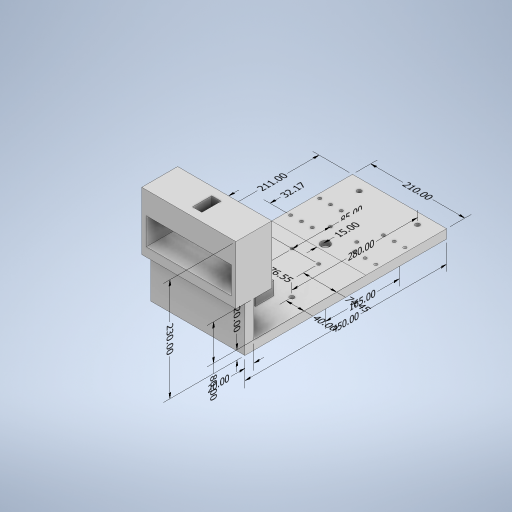
# Autodesk Inventor part: base
Saved by Autodesk Inventor 2023 (Build 270158000, 158)
## iProperties
Created: 2022-07-03
Part Number: base
Material: Genérico
Document SubType Name: Modeling
Designer: inigo
Density: 1 g/cm^3
Appearance: Valor por defecto
Author: inigo
Autodesk Inventor part; units mm, degrees
ref_plane "YZ Plane" through (0, 0, 0) normal (1, 0, 0) x (0, 1, 0)
ref_plane "XZ Plane" through (0, 0, 0) normal (0, 1, 0) x (-1, 0, 0)
ref_plane "XY Plane" through (0, 0, 0) normal (0, 0, 1) x (1, 0, 0)
sketch "Boceto1" plane through (0, 0, 0) normal (1, 0, 0) x (0, 1, 0)
  line L0 (10, 225) -> (-10, 225)
  line L1 (-10, 225) -> (-10, -225)
  line L2 (-10, -225) -> (10, -225)
  line L3 (10, -225) -> (10, 225)
  line L4 (10, 225) -> (-10, -225) construction
  line L5 (-10, 225) -> (10, -225) construction
  point P0 (0, 0)
  dimension "d0" = 20
  dimension "d1" = 450
  constraints: 12 end point, 2 midpoint, 2 parallel, 1 horizontal, 1 perpendicular
  measures "d0" distance of L2.end L1.end
  measures "d1" distance of L1.end L0.end
extrude "Extrusión1" add sketch "Boceto1" along normal blind 210
sketch "Boceto2" plane through (0, 10, 225) normal (0, 1, 0) x (1, 0, 0)
  line L0 (0, 0) -> (0, 450) projected
  line L1 (210, 0) -> (210, 450) projected
  line L2 (0, 0) -> (210, 0)
  line L3 (210, 0) -> (210, 20)
  line L4 (210, 20) -> (0, 20)
  line L5 (0, 20) -> (0, 0)
  point P0 (0, 225)
  dimension "d4" = 20
  constraints: 8 end point, 2 parallel, 1 horizontal, 1 perpendicular, 1 point on line
  measures "d4" distance of L3.end L2.end
extrude "Extrusión2" add sketch "Boceto2" along normal blind 80
sketch "Boceto3" plane through (0, 90, 225) normal (0, 1, 0) x (1, 0, 0)
  line L0 (0, 0) -> (210, 0) projected
  line L1 (0, 0) -> (210, 0)
  line L2 (210, 0) -> (210, -20)
  line L3 (210, -20) -> (0, -20)
  line L4 (0, -20) -> (0, 0)
  line L5 (0, 0) -> (210, 0)
  line L6 (210, 0) -> (210, 60)
  line L7 (210, 60) -> (0, 60)
  line L8 (0, 60) -> (0, 0)
  point P0 (0, 225)
  dimension "d7" = 20
  dimension "d8" = 210
  dimension "d9" = 60
  constraints: 16 end point, 4 parallel, 2 horizontal, 2 perpendicular
  measures "d7" distance of L1.end L2.end
  measures "d8" distance of L7.end L6.end
  measures "d9" distance of L6.end L5.end
extrude "Extrusión3" add sketch "Boceto3" along normal blind 130
sketch "Boceto4" plane through (0, 90, 245) normal (0, 0, 1) x (1, 0, 0)
  line L0 (10, 80) -> (200, 80)
  line L1 (200, 80) -> (200, 20)
  line L2 (200, 20) -> (10, 20)
  line L3 (10, 20) -> (10, 80)
  point P0 (0, -90)
  point P1 (0, 130)
  point P2 (210, 0)
  dimension "d12" = 190
  dimension "d13" = 60
  constraints: 8 end point, 2 parallel, 1 horizontal, 1 perpendicular
  measures "d12" distance of L1.end L2.end
  measures "d13" distance of L0.end L1.end
extrude "Extrusión4" cut sketch "Boceto4" against normal blind 60
sketch "Boceto5" plane through (0, 220, 225) normal (0, 1, 0) x (1, 0, 0)
  line L0 (94.5, -1.5) -> (115.5, -1.5)
  line L1 (115.5, -1.5) -> (115.5, 41.5)
  line L2 (115.5, 41.5) -> (94.5, 41.5)
  line L3 (94.5, 41.5) -> (94.5, -1.5)
  line L4 (94.5, -1.5) -> (115.5, 41.5) construction
  line L5 (115.5, -1.5) -> (94.5, 41.5) construction
  point P0 (0, 225)
  point P1 (105, 20)
  dimension "d18" = 21
  dimension "d19" = 43
  constraints: 12 end point, 2 midpoint, 2 parallel, 1 horizontal, 1 perpendicular
  measures "d18" distance of L2.end L1.end
  measures "d19" distance of L1.end L0.end
extrude "Extrusión5" cut sketch "Boceto5" against normal blind 43
sketch "Boceto6" plane through (0, 10, -225) normal (0, 1, 0) x (1, 0, 0)
  circle A0 centre (40, -305) radius 5
  circle A1 centre (40, -25) radius 5
  circle A2 centre (170, -305) radius 5
  circle A3 centre (170, -25) radius 5
  line L0 (0, -470) -> (210, -470) projected
  line L1 (0, 0) -> (210, 0) projected
  line L2 (0, 0) -> (0, -430) projected
  line L3 (210, 0) -> (210, -430) projected
  point P0 (0, -225)
  dimension "d23" = 10
  dimension "d24" = 10
  dimension "d25" = 10
  dimension "d26" = 10
  dimension "d27" = 165
  dimension "d28" = 25
  dimension "d29" = 25
  dimension "d30" = 165
  dimension "d31" = 40
  dimension "d32" = 40
  dimension "d33" = 40
  dimension "d34" = 40
  constraints: 4 centre point
  measures "d23" diameter of A0
  measures "d24" diameter of A1
  measures "d25" diameter of A2
  measures "d26" diameter of A3
  measures "d27" distance from line of L0 A0.centre
  measures "d28" distance from line of L1 A1.centre
  measures "d29" distance from line of L1 A3.centre
  measures "d30" distance from line of L0 A2.centre
  measures "d31" distance from line of L2 A0.centre
  measures "d32" distance from line of L2 A1.centre
  measures "d33" distance from line of L3 A3.centre
  measures "d34" distance from line of L3 A2.centre
extrude "Extrusión6" cut sketch "Boceto6" against normal blind 43
sketch "Boceto7" plane through (0, 10, -225) normal (0, 1, 0) x (1, 0, 0)
  line L0 (0, 0) -> (210, 0) projected
  line L1 (0, 0) -> (210, 0)
  line L2 (210, 0) -> (105, 0)
  line L3 (210, -390) -> (0, -390) projected
  line L4 (105, -390) -> (105, 0)
  circle A0 centre (40, -305) radius 5 projected
  circle A1 centre (40, -25) radius 5 projected
  line L5 (40, -305) -> (40, -25)
  line L6 (40, -165) -> (169.1036, -165)
  circle A2 centre (104.5518, -165) radius 10
  point P0 (0, -225)
  dimension "d44" = 20
  constraints: 10 end point, 4 midpoint, 2 horizontal, 1 centre point, 1 perpendicular
  measures "d44" diameter of A2
extrude "Extrusión7" cut sketch "Boceto7" against normal blind 10 contours A2 L6 L4 | L4 L6 A2 | L6 A2 L4 | L4 A2 L6
sketch "Boceto8" plane through (0, 10, -225) normal (0, 1, 0) x (1, 0, 0)
  circle A0 centre (104.5518, -165) radius 10 projected
  circle A1 centre (135.5518, -211) radius 3.5
  line L0 (104.5518, -165) -> (126.1125, -165)
  circle A2 centre (135.5518, -126) radius 3.5
  circle A3 centre (76.5518, -126) radius 3.5
  circle A4 centre (76.5518, -211) radius 3.5
  point P0 (0, -225)
  dimension "d51" = 7
  dimension "d52" = 7
  dimension "d54" = 7
  constraints: 4 centre point, 2 end point, 1 horizontal
  measures "d51" diameter of A1
  measures "d52" diameter of A2
  measures "d54" diameter of A4
extrude "Extrusión8" cut sketch "Boceto8" against normal blind 20 contours A1 | A2 | A3 | A4
sketch "Boceto9" plane through (0, 10, -225) normal (0, 1, 0) x (1, 0, 0)
  line L0 (0, -430) -> (210, -430) projected
  line L1 (0, -430) -> (210, -430)
  circle A0 centre (93.5, -410) radius 3
  line L2 (210, -430) -> (0, -430)
  circle A1 centre (116.5, -410) radius 3
  circle A2 centre (93.5, -380) radius 3
  circle A3 centre (116.5, -380) radius 3
  point P0 (0, -225)
  dimension "d59" = 20
  dimension "d64" = 20
  dimension "d65" = 30
  dimension "d66" = 30
  constraints: 4 centre point, 4 end point, 1 collinear
  measures "d59" distance from line of L0 A0.centre
  measures "d64" distance from line of A1.centre L0
  measures "d65" distance between centres of A3 A1
  measures "d66" distance of A2.centre A0.centre
extrude "Extrusión9" cut sketch "Boceto9" against normal blind 20
sketch "Boceto10" plane through (0, 10, -225) normal (0, 1, 0) x (1, 0, 0)
  line L0 (0, -430) -> (210, -430) projected
  line L1 (68, -358.4637) -> (142, -358.4637)
  line L2 (142, -358.4637) -> (68, -358.4637)
  line L3 (68, -358.4637) -> (68, -327.4637)
  line L4 (68, -327.4637) -> (142, -327.4637)
  line L5 (142, -327.4637) -> (142, -358.4637)
  line L6 (68, -358.4637) -> (142, -327.4637)
  line L7 (68, -327.4637) -> (142, -358.4637)
  line L8 (63, -363.4637) -> (147, -363.4637)
  line L9 (147, -363.4637) -> (147, -322.4637)
  line L10 (147, -322.4637) -> (63, -322.4637)
  line L11 (63, -322.4637) -> (63, -363.4637)
  line L12 (63, -363.4637) -> (147, -322.4637) construction
  line L13 (147, -363.4637) -> (63, -322.4637) construction
  point P0 (0, -225)
  point P1 (105, -342.9637)
  dimension "d68" = 74
  dimension "d69" = 31
  dimension "d70" = 84
  dimension "d71" = 41
  constraints: 26 end point, 4 parallel, 3 midpoint, 2 horizontal, 2 perpendicular
  measures "d68" distance of L1.start L1.end
  measures "d69" distance of L2.end L3.end
  measures "d70" distance of L10.end L9.end
  measures "d71" distance of L9.end L8.end
extrude "Extrusión10" cut sketch "Boceto10" against normal blind 10 contours L6 L7 L1 | L3 L7 L6 | L7 L6 L5 | L4 L6 L7
sketch "Boceto11" plane through (0, 10, -225) normal (0, 1, 0) x (1, 0, 0)
  line L0 (142, -358.4637) -> (68, -358.4637) projected
  line L1 (68, -358.4637) -> (142, -327.4637)
  line L2 (68, -327.4637) -> (142, -327.4637) projected
  line L3 (142, -327.4637) -> (68, -327.4637)
  line L4 (142, -327.4637) -> (142, -358.4637) projected
  line L5 (68, -327.4637) -> (142, -358.4637)
  line L6 (63, -363.4637) -> (147, -363.4637)
  line L7 (147, -363.4637) -> (147, -322.4637)
  line L8 (147, -322.4637) -> (63, -322.4637)
  line L9 (63, -322.4637) -> (63, -363.4637)
  line L10 (63, -363.4637) -> (147, -322.4637) construction
  line L11 (147, -363.4637) -> (63, -322.4637) construction
  line L12 (68, -358.4637) -> (142, -358.4637)
  line L13 (142, -358.4637) -> (142, -327.4637)
  line L14 (142, -327.4637) -> (68, -327.4637)
  line L15 (68, -327.4637) -> (68, -358.4637)
  line L16 (68, -358.4637) -> (142, -327.4637) construction
  line L17 (142, -358.4637) -> (68, -327.4637) construction
  point P0 (0, -225)
  point P1 (105, -342.9637)
  dimension "d74" = 84
  dimension "d75" = 41
  constraints: 30 end point, 5 equal length, 5 midpoint, 2 horizontal, 2 perpendicular
  measures "d74" distance of L8.end L7.end
  measures "d75" distance of L7.end L6.end
extrude "Extrusión11" add sketch "Boceto11" along normal blind 30
sketch "Boceto12" plane through (0, 10, -225) normal (0, 1, 0) x (1, 0, 0)
  circle A0 centre (10, -147.8334) radius 3.5
  line L0 (0, -155.4334) -> (68, -155.4334)
  line L1 (68, -155.4334) -> (68, -75.4334)
  line L2 (68, -75.4334) -> (0, -75.4334)
  line L3 (0, -75.4334) -> (0, -155.4334)
  line L4 (34, -155.4334) -> (34, -124.7606)
  circle A1 centre (34, -147.8334) radius 3.5
  circle A2 centre (58, -147.8334) radius 3.5
  line L5 (68, -115.4334) -> (56.8167, -115.4334)
  circle A3 centre (10, -83.0334) radius 3.5
  circle A4 centre (34, -83.0334) radius 3.5
  circle A5 centre (58, -83.0334) radius 3.5
  line L6 (0, 0) -> (210, 0) projected
  line L7 (105, 0) -> (105, -79.7219)
  circle A6 centre (200, -147.8334) radius 3.5
  line L8 (210, -155.4334) -> (142, -155.4334)
  line L9 (142, -155.4334) -> (142, -75.4334)
  line L10 (142, -75.4334) -> (210, -75.4334)
  line L11 (210, -75.4334) -> (210, -155.4334)
  line L12 (176, -155.4334) -> (176, -124.7606)
  circle A7 centre (176, -147.8334) radius 3.5
  circle A8 centre (152, -147.8334) radius 3.5
  line L13 (142, -115.4334) -> (153.1833, -115.4334)
  circle A9 centre (152, -83.0334) radius 3.5
  circle A10 centre (176, -83.0334) radius 3.5
  circle A11 centre (200, -83.0334) radius 3.5
  point P0 (0, -225)
  point P1 (210, -225)
  dimension "d78" = 7
  dimension "d79" = 68
  dimension "d80" = 80
  dimension "d81" = 7.6
  dimension "d82" = 10
  dimension "d83" = 7
  constraints: 26 end point, 12 centre point, 5 symmetric about line, 3 midpoint, 2 horizontal, 2 parallel, 2 point on line, 2 vertical, 1 perpendicular, 4 other
  measures "d78" diameter of A0
  measures "d79" distance of L2.end L1.end
  measures "d80" distance of L1.end L0.end
  measures "d81" distance from line of L0 A0.centre
  measures "d82" distance from line of L3 A0.centre
  measures "d83" diameter of A1
extrude "Extrusión12" cut sketch "Boceto12" against normal blind 30 contours A0 | A1 L4 | L4 A1 | A2 | A3 | A4 | A5 | A6 | A7 L12 | L12 A7 | A8 | A9 | A10 | A11
sketch "Boceto13" plane through (0, 10, -225) normal (0, 1, 0) x (1, 0, 0)
  line L0 (0, 0) -> (0, -430) projected
  line L1 (0, -180) -> (209.4793, -180)
  line L2 (0, 0) -> (210, 0) projected
  line L3 (0, -450) -> (0, 0) projected
  line L4 (0, -270) -> (210, -270)
  line L5 (210, -450) -> (210, 0) projected
  line L6 (210, -430) -> (0, -430) projected
  line L7 (0, -450) -> (210, -450) projected
  point P0 (0, -225)
  dimension "d103" = 180
  dimension "d110" = 180
  constraints: 4 end point, 3 point on line, 2 horizontal
  measures "d103" distance between parallel lines of L1 L2
  measures "d110" distance between parallel lines of L4 L7
split_face "Dividir1"
